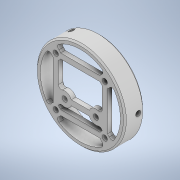
# Autodesk Inventor part: Elektro_Gyro
Saved by Autodesk Inventor 2020 (Build 240168000, 168)
## iProperties
Created: 2020-04-08
Part Number: Elektro_Gyro
Material: Generisch
Document SubType Name: Modeling
Designer: sp
Density: 1 g/cm^3
Appearance: Vorgabe
Author: sp
## iProperties of the stored document _3D-Druck.ipt
Created: 2020-04-15
Part Number: _3D-Druck
Material: Generisch
Document SubType Name: Modeling
Designer: sp
Density: 1 g/cm^3
Appearance: Vorgabe
Author: sp
Autodesk Inventor part; units mm, degrees
ref_plane "YZ Plane" through (0, 0, 0) normal (1, 0, 0) x (0, 1, 0)
ref_plane "XZ Plane" through (0, 0, 0) normal (0, 1, 0) x (-1, 0, 0)
ref_plane "XY Plane" through (0, 0, 0) normal (0, 0, 1) x (1, 0, 0)
sketch "Skizze1" plane through (0, 0, 0) normal (0, 0, 1) x (1, 0, 0)
  circle A0 centre (0, 0) radius 27
  circle A1 centre (0, 0) radius 30
  dimension "d0" = 54
  dimension "d1" = 60
  constraints: 2 centre point, 2 coincident
  measures "d0" diameter of A0
  measures "d1" diameter of A1
extrude "Extrusion1" add sketch "Skizze1" along normal mid plane 13
sketch "Skizze2" plane through (0, 0, 6.5) normal (0, 0, 1) x (1, 0, 0)
  line L0 (-43.452739, 16.5) -> (51.171113, 16.5) construction
  line L1 (-73.770433, -16.5) -> (86.29501, -16.5) construction
  line L2 (-73.770433, 0) -> (82.283344, 0) construction
  line L3 (0, 59.529809) -> (0, -61.622487) construction
  line L4 (16.5, 51.305895) -> (16.5, -53.398573) construction
  line L5 (-16.5, 51.305895) -> (-16.5, -45.776408) construction
  circle A0 centre (-16.5, 16.5) radius 1.75
  circle A1 centre (16.5, 16.5) radius 1.75
  circle A2 centre (16.5, -16.5) radius 1.75
  circle A3 centre (-16.5, -16.5) radius 1.75
  circle A4 centre (-16.5, 16.5) radius 3.680253
  circle A5 centre (16.5, 16.5) radius 3.689882
  circle A6 centre (16.5, -16.5) radius 3.665487
  circle A7 centre (-16.5, -16.5) radius 3.665674
  line L6 (14.123817, 14.75) -> (-13.823634, 14.75)
  line L7 (-13.823634, 14.75) -> (-13.823634, 18.25)
  line L8 (-13.823634, 18.25) -> (14.123817, 18.25)
  line L9 (14.123817, 18.25) -> (14.123817, 14.75)
  line L10 (-14.204856, -14.75) -> (14.123817, -14.75)
  line L11 (14.123817, -14.75) -> (14.123817, -18.25)
  line L12 (14.123817, -18.25) -> (-14.204856, -18.25)
  line L13 (-14.204856, -18.25) -> (-14.204856, -14.75)
  line L14 (14.75, 14.090792) -> (18.25, 14.090792)
  line L15 (18.25, 14.090792) -> (18.25, -14.061192)
  line L16 (18.25, -14.061192) -> (14.75, -14.061192)
  line L17 (14.75, -14.061192) -> (14.75, 14.090792)
  line L18 (-18.25, 14.090792) -> (-14.75, 14.090792)
  line L19 (-14.75, 14.090792) -> (-14.75, -14.061192)
  line L20 (-14.75, -14.061192) -> (-18.25, -14.061192)
  line L21 (-18.25, -14.061192) -> (-18.25, 14.090792)
  point P0 (0, 0)
  point P1 (-13.279027, -18.25)
  point P2 (13.27924, -18.25)
  point P3 (13.27924, -14.75)
  point P4 (-13.279027, -14.75)
  point P5 (13.251504, 18.25)
  point P6 (-13.262446, 18.25)
  point P7 (-13.262446, 14.75)
  point P8 (13.251504, 14.75)
  point P9 (18.25, 13.251504)
  point P10 (14.75, 13.251504)
  point P11 (14.75, -13.27924)
  point P12 (18.25, -13.27924)
  point P13 (-18.25, 13.262446)
  point P14 (-18.25, -13.279027)
  point P15 (-14.75, -13.279027)
  point P16 (-14.75, 13.262446)
  dimension "d4" = 33
  dimension "d5" = 33
  dimension "d6" = 3.5
  dimension "d7" = 3.5
  dimension "d8" = 3.5
  dimension "d9" = 3.5
  dimension "d10" = 3.5
  dimension "d11" = 3.5
  dimension "d13" = 3.5
  dimension "d14" = 3.5
  constraints: 44 end point, 10 point on line, 8 centre point, 8 parallel, 7 horizontal, 4 coincident, 4 perpendicular, 3 vertical, 6 other
  measures "d4" distance between parallel lines of L1 L0
  measures "d5" distance between parallel lines of L4 L5
  measures "d6" diameter of A0
  measures "d7" diameter of A1
  measures "d8" diameter of A2
  measures "d9" diameter of A3
  measures "d10" distance between parallel lines of L6 L8
  measures "d11" distance between parallel lines of L12 L10
  measures "d13" distance between parallel lines of L15 L17
  measures "d14" distance between parallel lines of L19 L21
extrude "Extrusion2" add sketch "Skizze2" against normal blind 3 contours A4 L6 L7 L8 | A4 L8 A5 L6 | L8 L7 L6 A4 L19 L18 L21 | L21 L18 L19 A4 | A4 L19 A7 L21 | L8 L9 L6 A5 | A5 L15 L14 L17 L6 L9 L8 | L21 L20 L19 A7 L10 L13 L12 | A7 L19 L20 L21 | L17 L14 L15 A5 | A5 L15 A6 L17 | L12 L13 L10 A7 | A7 L10 A6 L12 | L17 L16 L15 A6 L12 L11 L10 | A6 L15 L16 L17 | A6 L10 L11 L12
fillet "Rundung1" radius 2 8 edges at (19.4114, 18.7669, 5) (18.7669, 19.4114, 5) (-18.8397, 19.3408, 5) (-19.3408, 18.8397, 5) (-19.0629, -19.1208, 5) (-19.1208, -19.0629, 5) (19.0852, -19.0986, 5) (19.0986, -19.0852, 5)
sketch "Skizze3" plane through (0, 0, 0) normal (1, 0, 0) x (0, 1, 0)
  circle A0 centre (0, -2.5) radius 1.75
  line L0 (-30, -6.5) -> (30, -6.5) projected
  point P0 (0, 0)
  dimension "d18" = 3.5
  dimension "d19" = 4
  constraints: 1 centre point
  measures "d18" diameter of A0
  measures "d19" distance from line of L0 A0.centre
extrude "Extrusion3" cut sketch "Skizze3" along normal blind 30
pattern_circular "Runde Anordnung1" count 3 over 360 about axis through (0, 0, -10) along (0, 0, 1) of "Extrusion3"
chamfer "Fase1" distance 1 angle 45 2 edges at (-30, 0, 6.5) (-30, 0, -6.5)
sketch "Skizze5" plane through (0, 0, 6.5) normal (0, 0, 1) x (1, 0, 0)
  line L0 (14.75, -13.27924) -> (14.75, 13.251504)
  line L1 (-14.75, 13.262446) -> (-14.75, -13.279027)
  line L2 (14.75, -5.5) -> (-14.75, -5.5)
  line L3 (-14.75, -5.5) -> (-14.75, -9)
  line L4 (-14.75, -9) -> (14.75, -9)
  line L5 (14.75, -9) -> (14.75, -5.5)
  point P0 (0, 0)
  point P1 (-14.75, -5.5)
  dimension "d32" = 3.5
  dimension "d33" = 5.5
  constraints: 8 end point, 2 parallel, 2 point on line, 1 horizontal, 1 perpendicular
  measures "d32" distance of L3.end L2.end
  measures "d33" distance from line of point (0, 0) L2
extrude "Extrusion4" add sketch "Skizze5" against normal blind 3
sketch "Skizze4" plane through (0, 0, 6.5) normal (0, 0, 1) x (1, 0, 0)
  line L0 (0, 93.051445) -> (0, -93.051445) construction
  line L1 (44.274481, 0) -> (-44.274481, 0) construction
  line L2 (13.25, 9.75) -> (-13.25, 9.75) construction
  line L3 (-13.25, 9.75) -> (-13.25, -9.75) construction
  line L4 (-13.25, -9.75) -> (13.25, -9.75) construction
  line L5 (13.25, -9.75) -> (13.25, 9.75) construction
  line L6 (33.788288, -7.25) -> (-34.543316, -7.25) construction
  circle A0 centre (10.5, -7.25) radius 1.75
  circle A1 centre (10.5, -7.25) radius 4.75
  circle A2 centre (-10.5, -7.25) radius 1.75
  circle A3 centre (-10.5, -7.25) radius 4.75
  circle A4 centre (10.5, -7.25) radius 1.75
  circle A5 centre (-10.5, -7.25) radius 1.75
  point P0 (0, 0)
  point P1 (0, 0)
  dimension "d28" = 19.5
  dimension "d29" = 26.5
  dimension "d30" = 7.25
  dimension "d31" = 21
  dimension "d37" = 3.5
  dimension "d38" = 9.5
  dimension "d39" = 3.5
  dimension "d40" = 9.5
  dimension "d43" = 3.5
  dimension "d44" = 3.5
  constraints: 14 end point, 6 centre point, 6 coincident, 4 midpoint, 3 horizontal, 2 parallel, 2 point on line, 1 perpendicular, 1 symmetric about line, 1 vertical, 2 other
  measures "d28" distance of L4.end L2.start
  measures "d29" distance of L3.end L4.end
  measures "d30" distance between parallel lines of L1 L6
  measures "d31" distance of point (-10.5, -7.25) point (10.5, -7.25)
  measures "d37" diameter of A0
  measures "d38" diameter of A1
  measures "d39" diameter of A2
  measures "d40" diameter of A3
  measures "d43" diameter of A4
  measures "d44" diameter of A5
extrude "Extrusion5" add sketch "Skizze4" against normal blind 3
sketch "Skizze6" plane through (0, 0, 6.5) normal (0, 0, 1) x (1, 0, 0)
  arc A0 (14.75, -5.12868) -> (6.08412, -5.5) centre (10.5, -7.25) ccw
  circle A1 centre (10.5, -7.25) radius 1.75
  arc A2 (-14.75, -9.37132) -> (-6.08412, -9) centre (-10.5, -7.25) ccw
  circle A3 centre (-10.5, -7.25) radius 1.75
  point P0 (0, 0)
  point P1 (14.645781, -5.5)
  point P2 (-14.645781, -9)
  dimension "d45" = 3.5
  dimension "d46" = 3.5
  constraints: 2 centre point, 2 coincident
  measures "d45" diameter of A1
  measures "d46" diameter of A3
extrude "Extrusion6" cut sketch "Skizze6" against normal blind 3
fillet "Rundung2" radius 2 4 edges at (14.75, -9.3713, 5) (-14.75, -9.3713, 5) (-14.75, -5.1287, 5) (14.75, -5.1287, 5)
